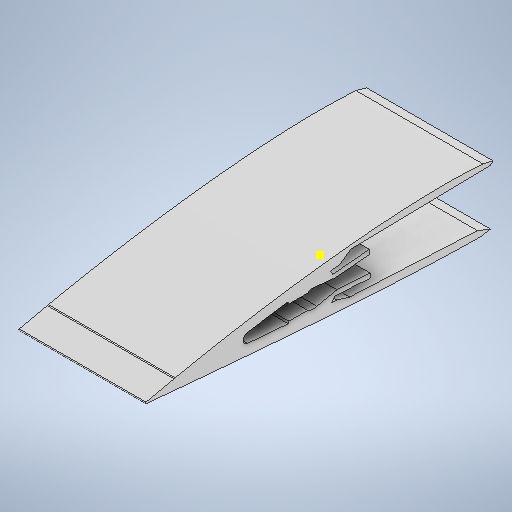
# Autodesk Inventor part: 1P.01.02.06-HB-Trailing adge access panel
Saved by Autodesk Inventor 2025.1 (Build 291241000, 241)
## iProperties
Created: 2025-01-16
Part Number: 1P.01.02.06-HB-Trailing adge access panel
Material: Generic
Document SubType Name: Modeling
Designer: hjbre
Density: 1 g/cm^3
Appearance: Default
Author: hjbre
Autodesk Inventor part; units mm, degrees
ref_plane "YZ Plane" through (0, 0, 0) normal (1, 0, 0) x (0, 1, 0)
ref_plane "XZ Plane" through (0, 0, 0) normal (0, 1, 0) x (-1, 0, 0)
ref_plane "XY Plane" through (0, 0, 0) normal (0, 0, 1) x (1, 0, 0)
sketch "Sketch1" plane through (0, 0, 0) normal (1, 0, 0) x (0, 1, 0)
  point P0 (0, 0)
sketch "Sketch2" plane through (0, -43.1688, 116.7453) normal (1, 0, 0) x (0, 0, -1)
  spline S0 degree 4 poles (254.4361, 38.2581) (252.1599, 38.6503) (246.7887, 39.4993) (237.9849, 40.6183) (225.3575, 41.7043) (211.2027, 42.3417) (196.3926, 42.4701) (181.0313, 42.0702) (165.5064, 41.2217) (149.7852, 40.0448) (134.1096, 38.5775) (118.6247, 36.8508) (103.5, 34.9393) (88.9016, 32.8834) (74.9958, 30.7382) (61.9178, 28.5627) (49.8271, 26.4098) (38.8354, 24.34) (29.0772, 22.4039) (20.6323, 20.6564) (13.6456, 19.1491) (6.9132, 17.6607) (2.9022, 16.74) (0.4691, 16.1882) (0, 16.065) knots 0.214297 0.214297 0.214297 0.214297 0.214297 0.24332 0.281775 0.321542 0.36238 0.404005 0.446178 0.488665 0.531231 0.573688 0.615803 0.657336 0.698047 0.737682 0.775986 0.812688 0.847495 0.880087 0.910093 0.937059 0.960363 1 1 1 1 1
  spline S1 degree 4 poles (300, 15.624) (299.8057, 13.313) (297.7085, 10.3432) (293.0509, 7.5008) (285.3959, 4.883) (278.1124, 3.2165) (269.5147, 1.8925) (259.681, 0.913) (248.7129, 0.2783) (236.7119, -0.0309) (223.8067, -0.0504) (210.1253, 0.1933) (195.7754, 0.645) (180.9677, 1.2494) (165.6517, 1.9825) (150.1916, 2.9048) (134.6873, 3.9451) (119.3375, 5.0495) (104.3042, 6.1987) (89.7566, 7.3561) (75.8492, 8.4887) (62.7429, 9.5824) (50.5811, 10.6226) (39.4971, 11.5797) (29.6294, 12.4513) (21.0711, 13.2264) (13.9642, 13.872) (7.1043, 14.5127) (2.9719, 14.899) (0.5336, 15.1402) (0, 15.183) knots 0 0 0 0 0 0.054374 0.079823 0.107915 0.138502 0.171346 0.206192 0.24279 0.280898 0.320285 0.360722 0.402033 0.443996 0.486385 0.528971 0.571474 0.613657 0.655281 0.696102 0.735871 0.774327 0.811194 0.846178 0.878951 0.909137 0.936275 0.959735 1 1 1 1 1
  arc A0 (0, 16.065) -> (0, 15.183) centre (0.1158, 15.624) ccw
  line L0 (0.1158, 15.624) -> (227.9902, 15.624) construction
  line L1 (300, 15.624) -> (0.1158, 15.624) construction
  line L2 (300, 15.624) -> (200, 15.624) construction
  line L3 (200, 15.624) -> (200, 42.3773) construction
  line L4 (200, 15.624) -> (200, 0.5273)
  line L5 (0, 0) -> (0, 20.241)
  line L6 (0, 20.241) -> (238.581, 20.241) construction
  circle A1 centre (238.581, 20.241) radius 14
  line L7 (238.581, 20.241) -> (208.581, 20.241)
  line L8 (238.581, 25.359) -> (238.581, 20.241)
  line L9 (0, 20.241) -> (112, 20.241)
  circle A2 centre (112, 20.241) radius 5.39
  line L10 (0, 15.624) -> (112, 15.624) construction
  line L11 (0, 15.624) -> (112, 15.624) construction
  line L12 (112, 15.624) -> (112, 35.9945)
  line L13 (112, 15.624) -> (112, 5.6153)
  line L14 (299.2071, 20.0822) -> (298.8742, 19.5363) construction
  arc A3 (298.904, 19.5932) -> (299.1702, 20.0296) centre (292.2911, 23.9254) ccw construction
  spline S2 degree 4 poles (299.2852, 20.241) (299.2279, 20.1316) (299.168, 20.0232) (299.1056, 19.9158) (299.0406, 19.8092) knots 0 0 0 0 0 1 1 1 1 1
  line L15 (299.432, 20.5214) -> (299.1384, 19.9606) construction
  arc A4 (299.1639, 20.0188) -> (299.3987, 20.4672) centre (292.801, 23.6361) ccw construction
  line L16 (294.5507, 15.7157) -> (294.2359, 15.5323) construction
  arc A5 (294.2672, 15.5511) -> (294.519, 15.6978) centre (283.8844, 33.657) ccw construction
  spline S3 degree 2 poles (295.8506, 16.56) (295.1573, 16.0692) (294.3933, 15.624) knots 0 0 0 1 1 1
  line L17 (295.9593, 16.4657) -> (295.7419, 16.6543) construction
  arc A6 (295.9374, 16.4843) -> (295.7635, 16.6352) centre (281.8729, 0.4516) ccw construction
  spline S4 degree 4 poles (296.8569, 15.624) (296.6183, 15.8629) (296.3707, 16.0985) (296.1147, 16.3309) (295.8506, 16.56) knots 0 0 0 0 0 1 1 1 1 1
  spline S5 degree 4 poles (219.5872, 34.9119) (218.6954, 34.952) (214.8585, 35.1063) (210.7072, 35.3295) (192.898, 35.4464) (181.4278, 35.0555) (165.1774, 34.1819) (149.5619, 33.1267) (133.8284, 31.3479) (128.2654, 31.0974) (123.3908, 30.59) knots 0 0 0 0 0 0.139244 0.23322 0.363937 0.509983 0.657115 0.798105 1 1 1 1 1
  line L18 (232.7438, 34.3645) -> (201.1936, 35.6815) construction
  arc A7 (229.5868, 34.4549) -> (204.3471, 35.5085) centre (136.3483, -1896.3245) ccw construction
  arc A8 (264.2661, 15.123) -> (264.3608, 15.624) centre (238.581, 20.241) ccw
  circle A9 centre (238.581, 20.241) radius 24
  circle A10 centre (112, 20.241) radius 15.39
  spline S6 degree 4 poles (300, 15.624) (300.2691, 17.9337) (298.7834, 21.2677) (294.6934, 24.9798) (287.5317, 28.9406) (280.4869, 31.8205) (271.481, 34.7182) (262.4868, 36.793) (257.7004, 37.6957) (254.4361, 38.2581) knots 0 0 0 0 0 0.247555 0.363857 0.49255 0.632996 0.778264 1 1 1 1 1
  line L19 (285.2945, 32.941) -> (223.5776, 43.5753) construction
  arc A11 (278.7224, 32.6349) -> (229.6682, 41.0872) centre (217.2184, -177.7386) ccw construction
  line L20 (285.2945, 32.941) -> (223.5776, 43.5753) construction
  arc A12 (278.8771, 33.0418) -> (229.6586, 41.5224) centre (200.8949, -272.4733) ccw construction
  line L21 (285.2945, 25.9322) -> (223.5776, 36.5664) construction
  spline S7 degree 4 poles (251.493, 31.7362) (243.7009, 32.9676) (232.1602, 34.2966) (216.4428, 35.2879) (196.3923, 35.4611) (181.0317, 35.0615) (165.5053, 34.2127) (149.7883, 33.0365) (134.1012, 31.5672) (118.6474, 29.8462) (103.4397, 27.9193) (89.0589, 25.9037) (74.8371, 23.6927) (62.4884, 21.6695) (49.6399, 19.3545) (46.3795, 18.7429) (43.8125, 18.259) knots 0 0 0 0 0 0.163963 0.232338 0.302031 0.372642 0.443778 0.515047 0.586134 0.656647 0.726187 0.794348 0.86071 0.920346 1 1 1 1 1
  line L22 (285.2945, 25.9322) -> (223.5776, 36.5664) construction
  arc A13 (278.7224, 25.626) -> (229.6682, 34.0784) centre (217.2184, -184.7474) ccw construction
  spline S8 degree 4 poles (295.845, 16.556) (295.7198, 16.6646) (294.585, 17.6283) (292.0585, 19.4283) (287.5167, 21.9347) (280.467, 24.8321) (271.9714, 27.5226) (264.2087, 29.4004) (258.4092, 30.5515) (255.0536, 31.1429) (254.4361, 31.2493) (253.9689, 31.3298) (253.5018, 31.4103) (253.0347, 31.4908) (252.5676, 31.5712) knots 0 0 0 0 0 0.018905 0.168959 0.334999 0.516204 0.711161 0.918337 0.964832 0.964832 0.964832 0.964832 1 1 1 1 1
  line L23 (270.129, 9.1254) -> (275.129, 9.1254) construction
  line L24 (281.07, 24.4582) -> (286.07, 24.4582) construction
  line L25 (318.8214, -3.3673) -> (272.8686, 36.4793) construction
  arc A14 (303.2079, 0.552) -> (278.9595, 21.5782) centre (281.8576, 0.4252) ccw construction
  line L26 (68.4884, 16.1198) -> (19.1367, 20.3983) construction
  arc A15 (63.5515, 16.5281) -> (24.0702, 19.9509) centre (-819.8994, -9944.3712) ccw construction
  line L27 (21.7244, 20.2173) -> (21.2001, 20.2647) construction
  arc A16 (21.2525, 20.26) -> (21.672, 20.222) centre (898.6358, 9712.9556) ccw construction
  spline S9 degree 4 poles (295.8353, 16.5644) (293.4171, 14.8846) (288.4135, 12.6926) (280.7063, 10.6698) (269.511, 8.9398) (259.6826, 7.9632) (248.7122, 7.3273) (236.7121, 7.0186) (223.8065, 6.9989) (210.1254, 7.2427) (195.7753, 7.6944) (180.968, 8.2987) (165.6509, 9.032) (150.1939, 9.954) (134.681, 10.995) (119.3545, 12.0974) (104.259, 13.2519) (89.8748, 14.3954) (75.7524, 15.5471) (62.9065, 16.6165) (50.5107, 17.6776) (46.5166, 18.0246) (43.8125, 18.259) knots 0 0 0 0 0 0.084767 0.124025 0.166179 0.210904 0.257877 0.306788 0.35734 0.409241 0.462263 0.516122 0.570528 0.625186 0.679738 0.73388 0.787304 0.839697 0.89074 0.937143 1 1 1 1 1
  spline S10 degree 4 poles (21.4623, 20.241) (20.6227, 20.317) (20.124, 20.3622) (19.9191, 20.3809) (19.554, 20.414) knots 0 0 0 0 0 1 1 1 1 1
  line L28 (74.2541, 23.9969) -> (13.371, 12.5211) construction
  arc A17 (68.1759, 22.7939) -> (19.47, 13.6134) centre (1053.3901, -5337.891) ccw construction
  line L29 (133.5337, 10.9635) -> (115.8396, 12.0942) construction
  arc A18 (117.618, 12.0789) -> (131.7678, 11.1747) centre (141.027, 267.2384) ccw construction
  spline S11 degree 4 poles (218.4375, 7.1934) (217.6173, 7.2408) (213.8192, 7.4688) (209.5863, 6.8507) (192.5485, 7.9441) (181.1469, 8.163) (165.7461, 9.0283) (149.1424, 9.8801) (139.9777, 10.7519) (129.1073, 11.2464) (124.6867, 11.5289) knots 0 0 0 0 0 0.127631 0.213723 0.333628 0.467446 0.602621 0.738424 0.880395 0.880395 0.880395 0.880395 0.880395
  line L30 (140.665, 32.3881) -> (106.1166, 28.792) construction
  arc A19 (137.222, 31.4497) -> (109.679, 28.5828) centre (140.6225, -134.9596) ccw construction
  circle A20 centre (238.581, 20.241) radius 18
  line L31 (238.581, 38.241) -> (225.78, 41.559)
  line L32 (238.581, 2.241) -> (224.22, 0)
  line L33 (214.581, 20.241) -> (214.581, 42.1266) construction
  line L34 (127.39, 20.241) -> (127.39, 11.5255) construction
  line L35 (127.39, 20.241) -> (131.3139, 20.241) construction
  line L36 (96.61, 20.241) -> (96.61, 13.8631) construction
  line L37 (270.129, 5.6153) -> (270.129, 15.624) construction
  line L38 (272.129, 7.6153) -> (272.129, 13.624)
  line L39 (268.129, 13.624) -> (268.129, 7.6153)
  arc A21 (268.129, 7.6153) -> (272.129, 7.6153) centre (270.129, 7.6153) ccw
  arc A22 (272.129, 13.624) -> (268.129, 13.624) centre (270.129, 13.624) ccw
  line L40 (268.129, 24.172) -> (268.129, 30.1807)
  line L41 (270.129, 32.1807) -> (270.129, 22.172) construction
  arc A23 (272.129, 30.1807) -> (268.129, 30.1807) centre (270.129, 30.1807) ccw
  line L42 (272.129, 30.1807) -> (272.129, 24.172)
  arc A24 (268.129, 24.172) -> (272.129, 24.172) centre (270.129, 24.172) ccw
  arc A25 (200, 42.3155) -> (199.8538, 42.3773) centre (190.581, 20.241) ccw
  arc A26 (171.273, 34.4958) -> (171.2681, 34.4892) centre (190.581, 20.241) ccw
  arc A27 (210.7484, 7.2304) -> (209.2875, 35.2765) centre (190.581, 20.241) ccw
  arc A28 (169.4455, 8.8703) -> (169.4744, 8.8168) centre (190.581, 20.241) ccw
  arc A29 (153.9768, 9.6824) -> (154.0303, 9.7394) centre (142.78, 20.241) ccw
  arc A30 (151.2419, 33.0959) -> (151.2193, 33.1107) centre (142.78, 20.241) ccw
  arc A31 (132.1299, 31.3508) -> (130.3229, 11.2037) centre (142.78, 20.241) ccw
  arc A32 (95.2741, 13.9693) -> (95.1698, 26.7415) centre (81.22, 20.241) ccw
  arc A33 (66.334, 16.3348) -> (66.5389, 15.624) centre (81.22, 20.241) ccw
  circle A34 centre (112, 20.241) radius 6.205
  circle A35 centre (238.581, 20.241) radius 15.15
  line L43 (209.2875, 35.2765) -> (209.2875, 7.2282) construction
  line L44 (209.2875, 35.2765) -> (237.3358, 35.2765) construction
  line L45 (270.129, 22.172) -> (270.129, 15.624) construction
  arc A36 (207.7484, 7.2304) -> (206.2486, 35.3248) centre (187.581, 20.241) ccw
  spline S12 degree 4 poles (211.3665, 32.2395) (210.8467, 32.2487) (210.327, 32.2579) (209.8072, 32.2671) (209.2875, 32.2763) (209.0495, 32.2805) (208.8115, 32.2847) (208.5734, 32.2889) (208.3354, 32.2931) (207.2123, 32.313) (202.6658, 32.3768) (191.8163, 32.4121) (181.353, 32.0555) (165.1027, 31.1819) (149.4871, 30.1267) (133.7537, 28.3479) (128.1907, 28.0974) (123.316, 27.59) knots 0.151979 0.151979 0.151979 0.151979 0.151979 0.174428 0.174428 0.174428 0.174428 0.184709 0.184709 0.184709 0.184709 0.23322 0.363937 0.509983 0.657115 0.798105 1 1 1 1 1
  line L46 (215.7946, 32.1611) -> (200.8762, 32.4252) construction
  arc A37 (214.3012, 32.1394) -> (202.368, 32.3508) centre (201.7734, -338.2842) ccw construction
  line L47 (133.5153, 13.9635) -> (115.8212, 15.0942) construction
  arc A38 (117.5996, 15.0789) -> (131.7494, 14.1747) centre (141.0085, 270.2384) ccw construction
  spline S13 degree 4 poles (209.3847, 10.2111) (207.9788, 10.2003) (203.4382, 10.2427) (192.0384, 10.9536) (181.1285, 11.163) (165.7277, 12.0283) (149.124, 12.8801) (139.9593, 13.7519) (129.0889, 14.2464) (124.6682, 14.5289) knots 0.148112 0.148112 0.148112 0.148112 0.148112 0.213723 0.333628 0.467446 0.602621 0.738424 0.880395 0.880395 0.880395 0.880395 0.880395
  line L48 (216.9051, 10.269) -> (201.8643, 10.1532) construction
  arc A39 (203.3787, 10.3523) -> (215.3878, 10.4448) centre (208.6432, 106.4922) ccw construction
  line L49 (168.2894, 34.3211) -> (168.2894, 8.8793)
  line L50 (171.2681, 34.4892) -> (171.2681, 8.7233)
  line L51 (172.4463, 33.1033) -> (211.5485, 10.663)
  line L52 (170.8103, 30.2526) -> (209.9125, 7.8123)
  line L53 (205.1136, 34.0978) -> (138.1138, 30.2526)
  line L54 (138.1138, 30.2526) -> (137.8255, 35.2765)
  line L55 (137.8255, 35.2765) -> (205.1136, 39.1382)
  line L56 (205.1136, 34.0978) -> (205.1136, 39.1382)
  line L57 (205.1136, 34.0978) -> (210.154, 34.0978) construction
  line L58 (209.3931, 30.2526) -> (218.4375, 30.2526)
  line L59 (218.4375, 30.2526) -> (218.4375, 20.241)
  line L60 (218.4375, 10.2294) -> (218.4375, 20.241)
  line L61 (210.7484, 10.2294) -> (218.4375, 10.2294)
  line L62 (205.1136, 10.2653) -> (205.1136, 1.3438)
  line L63 (137.8255, 5.2055) -> (205.1136, 1.3438)
  line L64 (138.3156, 13.7456) -> (137.8255, 5.2055)
  line L65 (218.0871, 32.1205) -> (200.4879, 32.4321) construction
  arc A40 (202.2479, 32.4034) -> (216.3272, 32.1541) centre (386.3359, 10030.7089) ccw construction
  line L66 (127.39, 20.241) -> (125.0989, 20.241)
  line L67 (125.0989, 20.241) -> (125.0989, 30.1807)
  line L68 (125.0989, 30.1807) -> (127.39, 30.1807)
  line L69 (127.39, 30.1807) -> (127.39, 20.241)
  line L70 (127.39, 11.3668) -> (127.39, 20.241)
  line L71 (125.0989, 20.241) -> (125.0989, 11.5029)
  line L72 (215.7946, 29.1611) -> (200.8762, 29.4252) construction
  line L73 (218.0871, 29.1205) -> (200.4879, 29.4321) construction
  arc A41 (214.3012, 29.1394) -> (202.368, 29.3508) centre (201.7734, -341.2842) ccw construction
  arc A42 (202.2479, 29.4034) -> (216.3272, 29.1541) centre (386.3359, 10027.7089) ccw construction
  spline S14 degree 4 poles (211.3665, 29.2395) (210.8467, 29.2487) (210.327, 29.2579) (209.8072, 29.2671) (209.2875, 29.2763) (209.0495, 29.2805) (208.8115, 29.2847) (208.5734, 29.2889) (208.3354, 29.2931) (207.2123, 29.313) (202.6658, 29.3768) (191.8163, 29.4121) (181.353, 29.0555) (165.1027, 28.1819) (149.4871, 27.1267) (133.7537, 25.3479) (128.1907, 25.0974) (123.316, 24.59) knots 0.151979 0.151979 0.151979 0.151979 0.151979 0.174428 0.174428 0.174428 0.174428 0.184709 0.184709 0.184709 0.184709 0.23322 0.363937 0.509983 0.657115 0.798105 1 1 1 1 1
  line L74 (133.5153, 16.9635) -> (115.8212, 18.0942) construction
  line L75 (216.9051, 13.269) -> (201.8643, 13.1532) construction
  arc A43 (117.5996, 18.0789) -> (131.7494, 17.1747) centre (141.0085, 273.2384) ccw construction
  arc A44 (203.3787, 13.3523) -> (215.3878, 13.4448) centre (208.6432, 109.4922) ccw construction
  spline S15 degree 4 poles (209.3847, 13.2111) (207.9788, 13.2003) (203.4382, 13.2427) (192.0384, 13.9536) (181.1285, 14.163) (165.7277, 15.0283) (149.124, 15.8801) (139.9593, 16.7519) (129.0889, 17.2464) (124.6682, 17.5289) knots 0.148112 0.148112 0.148112 0.148112 0.148112 0.213723 0.333628 0.467446 0.602621 0.738424 0.880395 0.880395 0.880395 0.880395 0.880395
  line L76 (149.7183, 29.984) -> (149.7183, 26.984)
  line L77 (150.1886, 12.928) -> (150.1886, 15.928)
  line L78 (128.0727, 24.7738) -> (112, 26.446)
  line L79 (128.8956, 17.5289) -> (112, 14.036)
  line L80 (135.213, 15.013) -> (136.481, 8.8793)
  line L81 (135.213, 25.469) -> (137.9914, 38.9085)
  line L82 (112, 25.2109) -> (94.8048, 25.2109)
  line L83 (94.8048, 25.2109) -> (94.8048, 15.2109)
  line L84 (94.8048, 15.2109) -> (112, 15.2109)
  line L85 (112, 15.2109) -> (112, 25.2109)
  line L86 (230.4684, 4.1728) -> (136.481, 8.8793)
  line L87 (230.4684, 4.1728) -> (230.4684, 36.3092)
  line L88 (137.454, 36.3092) -> (128.0727, 29.984)
  line L89 (136.481, 8.8793) -> (127.39, 11.5255)
  line L90 (230.4684, 36.3092) -> (230.4684, 38.0731)
  line L91 (230.4684, 38.0731) -> (137.454, 36.3092)
  line L92 (230.4684, 38.0731) -> (232.7265, 39.7585)
  line L93 (222.1301, 4.5904) -> (230.9487, 1.05)
  point P0 (0.783, 16.254)
  point P1 (3.213, 16.812)
  point P2 (7.239, 17.724)
  point P3 (12.813, 18.96)
  point P4 (19.884, 20.484)
  point P5 (28.374, 22.245)
  point P6 (38.199, 24.195)
  point P7 (49.254, 26.28)
  point P8 (61.419, 28.446)
  point P9 (74.571, 30.636)
  point P10 (88.56, 32.793)
  point P11 (103.242, 34.86)
  point P12 (118.455, 36.783)
  point P13 (134.028, 38.511)
  point P14 (149.793, 39.984)
  point P15 (165.576, 41.16)
  point P16 (181.206, 41.985)
  point P17 (196.638, 42.363)
  point P18 (211.554, 42.222)
  point P19 (239.145, 40.389)
  point P20 (262.68, 36.666)
  point P21 (272.577, 34.218)
  point P22 (281.07, 31.467)
  point P23 (288.069, 28.491)
  point P24 (293.505, 25.359)
  point P25 (297.324, 22.137)
  point P26 (300, 15.624)
  point P27 (0.861, 15.105)
  point P28 (3.342, 14.868)
  point P29 (7.446, 14.481)
  point P30 (13.122, 13.953)
  point P31 (20.31, 13.296)
  point P32 (28.92, 12.519)
  point P33 (38.856, 11.64)
  point P34 (50.007, 10.674)
  point P35 (62.244, 9.63)
  point P36 (75.429, 8.529)
  point P37 (89.418, 7.389)
  point P38 (104.052, 6.228)
  point P39 (119.172, 5.076)
  point P40 (134.613, 3.966)
  point P41 (150.207, 2.928)
  point P42 (165.783, 2.013)
  point P43 (181.167, 1.263)
  point P44 (196.068, 0.663)
  point P45 (210.468, 0.225)
  point P46 (237.189, 0.039)
  point P47 (249.246, 0.378)
  point P48 (260.262, 1.05)
  point P49 (270.129, 2.076)
  point P50 (278.739, 3.462)
  point P51 (285.993, 5.211)
  point P52 (291.81, 7.314)
  point P53 (296.121, 9.756)
  point P54 (298.863, 12.531)
  point P55 (200, 15.624)
  point P56 (225.3642, 15.624)
  point P57 (238.581, 6.241)
  point P58 (238.581, 34.241)
  point P59 (225.3642, 15.624)
  point P60 (251.7978, 15.624)
  point P61 (0, 16.065)
  point P62 (0, 15.183)
  point P63 (224.581, 20.241)
  point P64 (112, 14.851)
  point P65 (112, 25.631)
  point P66 (0, 9.065)
  point P67 (0.783, 9.254)
  point P68 (3.213, 9.812)
  point P69 (7.239, 10.724)
  point P70 (12.813, 11.96)
  point P71 (19.884, 13.484)
  point P72 (28.374, 15.245)
  point P73 (38.199, 17.195)
  point P74 (49.254, 19.28)
  point P75 (61.419, 21.446)
  point P76 (74.571, 23.636)
  point P77 (88.56, 25.793)
  point P78 (103.242, 27.86)
  point P79 (118.455, 29.783)
  point P80 (134.028, 31.511)
  point P81 (149.793, 32.984)
  point P82 (165.576, 34.16)
  point P83 (181.206, 34.985)
  point P84 (225.78, 34.559)
  point P85 (239.145, 33.389)
  point P86 (251.493, 31.745)
  point P87 (262.68, 29.666)
  point P88 (272.577, 27.218)
  point P89 (281.07, 24.467)
  point P90 (288.069, 21.491)
  point P91 (293.505, 18.359)
  point P92 (297.324, 15.137)
  point P93 (299.493, 11.879)
  point P94 (300, 8.624)
  point P95 (-0.0042, 22.1841)
  point P96 (0.861, 22.105)
  point P97 (3.342, 21.868)
  point P98 (7.446, 21.481)
  point P99 (13.122, 20.953)
  point P100 (20.31, 20.296)
  point P101 (28.92, 19.519)
  point P102 (38.856, 18.64)
  point P103 (50.007, 17.674)
  point P104 (62.244, 16.63)
  point P105 (75.429, 15.529)
  point P106 (89.418, 14.389)
  point P107 (104.052, 13.228)
  point P108 (119.172, 12.076)
  point P109 (134.613, 10.966)
  point P110 (150.207, 9.928)
  point P111 (165.783, 9.013)
  point P112 (181.167, 8.263)
  point P113 (196.068, 7.663)
  point P114 (210.468, 7.225)
  point P115 (224.22, 7)
  point P116 (237.189, 7.039)
  point P117 (249.246, 7.378)
  point P118 (260.262, 8.05)
  point P119 (270.129, 9.076)
  point P120 (278.739, 10.462)
  point P121 (285.993, 12.211)
  point P122 (291.81, 14.314)
  point P123 (296.121, 16.756)
  point P124 (298.863, 19.531)
  point P125 (300, 22.624)
  point P126 (18.7405, 20.241)
  point P127 (216.9687, 35.023)
  point P128 (0, 16.065)
  point P129 (296.8569, 15.624)
  point P130 (294.3933, 15.624)
  point P131 (219.5872, 34.9119)
  point P132 (123.3908, 30.59)
  point P133 (254.4361, 38.2581)
  point P134 (0, 9.0562)
  point P135 (0.783, 9.2452)
  point P136 (3.213, 9.8032)
  point P137 (7.239, 10.7152)
  point P138 (12.813, 11.9512)
  point P139 (19.884, 13.4752)
  point P140 (28.374, 15.2362)
  point P141 (38.199, 17.1862)
  point P142 (49.254, 19.2712)
  point P143 (61.419, 21.4372)
  point P144 (74.571, 23.6272)
  point P145 (88.56, 25.7842)
  point P146 (103.242, 27.8512)
  point P147 (118.455, 29.7742)
  point P148 (134.028, 31.5022)
  point P149 (149.793, 32.9752)
  point P150 (165.576, 34.1512)
  point P151 (181.206, 34.9762)
  point P152 (196.638, 35.3542)
  point P153 (211.554, 35.2132)
  point P154 (225.78, 34.5502)
  point P155 (254.4361, 31.2493)
  point P156 (278.8769, 26.0734)
  point P157 (229.5906, 33.8662)
  point P158 (216.8848, -206.3625)
  point P159 (262.68, 29.6572)
  point P160 (272.577, 27.2092)
  point P161 (297.324, 15.1282)
  point P162 (299.493, 11.8702)
  point P163 (300, 8.6152)
  point P164 (-0.0042, 22.2335)
  point P165 (0.861, 22.1544)
  point P166 (3.342, 21.9174)
  point P167 (7.446, 21.5304)
  point P168 (13.122, 21.0024)
  point P169 (28.92, 19.5684)
  point P170 (38.856, 18.6894)
  point P171 (50.007, 17.7234)
  point P172 (62.244, 16.6794)
  point P173 (75.429, 15.5784)
  point P174 (89.418, 14.4384)
  point P175 (104.052, 13.2774)
  point P176 (119.172, 12.1254)
  point P177 (134.613, 11.0154)
  point P178 (150.207, 9.9774)
  point P179 (165.783, 9.0624)
  point P180 (181.167, 8.3124)
  point P181 (196.068, 7.7124)
  point P182 (210.468, 7.2744)
  point P183 (224.22, 7.0494)
  point P184 (237.189, 7.0884)
  point P185 (249.246, 7.4274)
  point P186 (260.262, 8.0994)
  point P187 (278.739, 10.5114)
  point P188 (285.993, 12.2604)
  point P189 (296.121, 16.8054)
  point P190 (298.863, 19.5804)
  point P191 (300, 22.6734)
  point P192 (225.7, -0.0094)
  point P193 (252.2617, 0.522)
  point P194 (227.3495, 41.4508)
  point P195 (105.9778, 6.0782)
  point P196 (115.8008, 5.3277)
  point P197 (98.26, 27.1738)
  point P198 (260.4522, 30.1228)
  point P199 (123.5853, 30.3718)
  dimension "d21" = 100
  dimension "d20" = 20.241
  dimension "d19" = 238.581
  dimension "d18" = 28
  dimension "d17" = 112
  dimension "d16" = 10.78
  dimension "d15" = 112
  dimension "d25" = 0
  dimension "d13" = 10
  dimension "d12" = 10
  dimension "d8" = 4
  dimension "d26" = 90
  dimension "d7" = 4
  dimension "d6" = 12.41
  dimension "d5" = 30.3
  dimension "d4" = 90
  dimension "d3" = 209.6276
  dimension "d2" = 270.4692
  dimension "d11" = 7.0088
  dimension "d9" = 7.0494
  dimension "d14" = 7
  dimension "d10" = 7.0494
  dimension "d1" = 6.548
  dimension "d0" = 90
  constraints: 191 end point, 83 point on circle, 48 midpoint, 45 centre point, 34 point on line, 14 perpendicular, 13 symmetric about line, 12 horizontal, 7 parallel, 7 tangent, 4 coincident, 3 collinear, 3 equal length, 3 vertical, 260 other
  measures "d21" distance of L1.start L2.end
  measures "d20" distance of L5.start L5.end
  measures "d19" distance of L5.end L6.end
  measures "d18" diameter of A1
  measures "d17" distance of L5.end L9.end
  measures "d16" diameter of A2
  measures "d15" distance of L10.start L10.end
  measures "d25" distance between parallel lines of L11 L10
  measures "d13" radial gap between concentric circles of A1 A9
  measures "d12" radial gap between concentric circles of A2 A10
  measures "d8" radial gap between concentric circles of A1 A20
  measures "d26" angle of L34 L35
  measures "d7" diameter of A22
  measures "d6" diameter of A34
  measures "d5" diameter of A35
  measures "d4" angle of L43 L44
  measures "d3" distance from line of point (-0.34, 15.624) L43
  measures "d2" horizontal distance of point (-0.34, 15.624) point (270.129, 18.898)
  measures "d11" distance of point (196.638, 35.354) point (196.638, 42.363)
  measures "d9" distance of point (196.068, 0.663) point (196.068, 7.712)
  measures "d14" distance of point (149.793, 32.984) point (149.793, 39.984)
  measures "d10" distance of point (150.207, 2.928) point (150.207, 9.977)
  measures "d1" distance of point (270.129, 15.624) point (270.129, 22.172)
  measures "d0" angle of L57 L56
extrude "Extrusion1" add sketch "Sketch2" against normal blind 85 contours L31 A9 L91 L56 L55 L81 S0 | L31 L92 L91 A9 | L81 L88 S5 A10 L12 S0 | L12 A10 S7 L9 S10 S0 | L91 L55 L56 | S10 L9 S0 | A10 S7 L12 | L12 S7 A10 | L88 S7 A10 S5 | L9 S7 S9 A10 S1 L5 S0 | S7 A10 L67 L78 A34 L12 | L12 A34 L82 A10 S7 | A10 L82 A32 S7 | L5 A0 | L81 S14 A31 S12 | S12 L76 S14 L81 | A31 S14 L69 S12 | S1 L4 L63 L62 L86 A9 L32 | A9 L86 L93 L32 | A10 S9 L13 S1 | L67 S12 A10 L78 | S12 L69 S14 L78 A10 | L84 A34 L13 S9 A10 | A10 S9 A32 L84 | S1 A10 S11 L89 L86 L64 L63 L4 | L13 S9 A10 S1 | L79 L71 A10 S9 L13 A34 | L63 L64 L86 L4 | L4 L86 L62 L63 | L79 A10 S13 L71 | S13 A10 L71 | L79 L70 S13 A10 | L77 S13 A31 L79 S15 | L79 A31 S13 L70
fillet "Fillet1" radius 3.175 1 edges at (-42.5, -24.9098, 72.9328)
body "Solid1"
